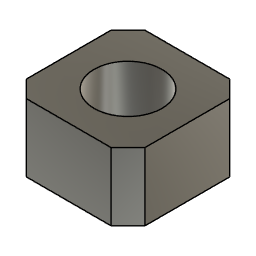
Base v1 (Autodesk Fusion 360 design; units mm, degrees)
Autodesk Fusion 360 part; units mm, degrees
sketch "Sketch1" plane through (0, 0, 0) normal (0, 0, 1) x (1, 0, 0)
  circle A0 centre (0, 0) radius 2
  line L0 (2.5, 3.5) -> (-2.5, 3.5)
  line L1 (-3.5, 2.5) -> (-3.5, -2.5)
  line L2 (-2.5, -3.5) -> (2.5, -3.5)
  line L3 (3.5, -2.5) -> (3.5, 2.5)
  line L4 (3.5, 3.5) -> (-3.5, -3.5) construction
  line L5 (-3.5, 3.5) -> (3.5, -3.5) construction
  line L6 (2.5, 3.5) -> (3.5, 2.5)
  line L7 (-2.5, 3.5) -> (-3.5, 2.5)
  line L8 (2.5, -3.5) -> (3.5, -2.5)
  line L9 (-2.5, -3.5) -> (-3.5, -2.5)
  dimension "d1" = 4
  dimension "d2" = 7
  dimension "d3" = 7
  dimension "d4" = 1
  dimension "d5" = 1
  dimension "d6" = 1
  dimension "d7" = 1
  dimension "d8" = 1
  dimension "d9" = 1
  dimension "d10" = 1
  dimension "d11" = 1
  constraint coincident A0.centre origin
  constraint horizontal L0
  constraint perpendicular L0 L1
  constraint parallel L0 L2
  constraint parallel L1 L3
  constraint coincident L4 A0.centre
  constraint coincident L5 A0.centre
  constraint coincident L4.start L0
  constraint coincident L4.start L3
  constraint coincident L5.start L0
  constraint coincident L5.start L1
  constraint coincident L5.end L2
  constraint coincident L5.end L3
  constraint coincident L4.end L2
  constraint coincident L4.end L1
  measures "d1" diameter of A0
  measures "d2" distance of L4.end L5.end
  measures "d3" distance of L5.start L4.end
  measures "d4" distance of L4.start L0.start
  measures "d5" distance of L4.start L3.end
  measures "d6" distance of L5.start L0.end
  measures "d7" distance of L5.start L1.start
  measures "d8" distance of L5.end L2.end
  measures "d9" distance of L5.end L3.start
  measures "d10" distance of L4.end L2.start
  measures "d11" distance of L4.end L1.end
extrude "Extrude1" add sketch "Sketch1" along normal blind 4
equation "d5 = d4"
equation "d7 = d6"
equation "d9 = d8"
equation "d11 = d10"
